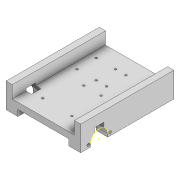
# Autodesk Inventor part: 본체판(구)
Saved by Autodesk Inventor 2020 (Build 240168000, 168)
## iProperties
Created: 2022-08-24
Part Number: 본체판(구)
Material: 일반
Document SubType Name: Modeling
Designer: 박연호
Density: 1 g/cm^3
Appearance: 기본값
Author: 박연호
Autodesk Inventor part; units mm, degrees
ref_plane "YZ Plane" through (0, 0, 0) normal (1, 0, 0) x (0, 1, 0)
ref_plane "XZ Plane" through (0, 0, 0) normal (0, 1, 0) x (-1, 0, 0)
ref_plane "XY Plane" through (0, 0, 0) normal (0, 0, 1) x (1, 0, 0)
sketch "스케치1" plane through (0, 0, 0) normal (0, 1, 0) x (-1, 0, 0)
  line L0 (60, 75) -> (-60, 75)
  line L1 (-60, 75) -> (-60, -75)
  line L2 (-60, -75) -> (60, -75)
  line L3 (60, -75) -> (60, 75)
  line L4 (60, 75) -> (-60, -75) construction
  line L5 (-60, 75) -> (60, -75) construction
  point P0 (0, 0)
  dimension "d0" = 120
  dimension "d1" = 150
  constraints: 12 end point, 2 midpoint, 2 parallel, 1 horizontal, 1 perpendicular
  measures "d0" distance of L0.start L0.end
  measures "d1" distance of L0.end L1.end
extrude "돌출1" add sketch "스케치1" along normal blind 40
sketch "스케치2" plane through (0, 40, 0) normal (0, 1, 0) x (1, 0, 0)
  line L0 (60, -75) -> (60, 75) projected
  line L1 (60, 75) -> (-60, 75) projected
  line L2 (50, 102.1646) -> (-50, 102.1646)
  line L3 (-50, 102.1646) -> (-50, -103.0725)
  line L4 (-50, -103.0725) -> (50, -103.0725)
  line L5 (50, -103.0725) -> (50, 102.1646)
  line L6 (-60, 75) -> (-60, -75) projected
  point P0 (0, 0)
  point P1 (50, 75)
  point P2 (-50, 75)
  dimension "d6" = 10
  dimension "d7" = 10
  constraints: 8 end point, 2 parallel, 1 horizontal, 1 perpendicular
  measures "d6" distance between parallel lines of L5 L0
  measures "d7" distance between parallel lines of L6 L3
extrude "돌출2" cut sketch "스케치2" against normal blind 20 contours L5 L4 L3 L1
sketch "스케치3" plane through (60, 0, 75) normal (1, 0, 0) x (0, 0, -1)
  circle A0 centre (29.6769, 5) radius 14
  circle A1 centre (120, 5) radius 14
  line L0 (150, 0) -> (150, 40) projected
  line L1 (0, 0) -> (150, 0) projected
  point P0 (75, 0)
  dimension "d10" = 28
  dimension "d12" = 28
  dimension "d13" = 30
  dimension "d16" = 5
  dimension "d30" = 5
  constraints: 2 centre point
  measures "d10" diameter of A0
  measures "d12" diameter of A1
  measures "d13" distance from line of L0 A1.centre
  measures "d16" distance from line of L1 A0.centre
  measures "d30" distance from line of L1 A1.centre
extrude "돌출3" cut sketch "스케치3" against normal blind 19 contours A0 L1 | L1 A0
sketch "스케치4" plane through (60, 0, -75) normal (1, 0, 0) x (0, 0, -1)
  arc A0 (-107.2464, 0) -> (-133.3998, 0) centre (-120.3231, 5) ccw projected
  line L0 (-134.3231, 36.9687) -> (-106.3231, 36.9687)
  line L1 (-106.3231, 36.9687) -> (-106.3231, -26.9687)
  line L2 (-106.3231, -26.9687) -> (-134.3231, -26.9687)
  line L3 (-134.3231, -26.9687) -> (-134.3231, 36.9687)
  line L4 (-134.3231, 36.9687) -> (-106.3231, -26.9687) construction
  line L5 (-106.3231, 36.9687) -> (-134.3231, -26.9687) construction
  line L6 (-150, 0) -> (-133.3998, 0) projected
  line L7 (-107.2464, 0) -> (0, 0) projected
  point P0 (-75, 0)
  point P1 (-134.3231, 0)
  point P2 (-134.3231, 5)
  point P3 (-106.3231, 0)
  point P4 (-106.3231, 5)
  dimension "d17" = 28
  constraints: 12 end point, 2 midpoint, 2 parallel, 1 horizontal, 1 perpendicular
  measures "d17" distance of L1.end L2.end
extrude "돌출4" cut sketch "스케치4" against normal blind 19 contours A0 L1 L7 | A0 L6 L3
sketch "스케치5" plane through (60, 0, -75) normal (1, 0, 0) x (0, 0, -1)
  line L0 (-127.8231, 12) -> (-112.8231, 12)
  line L1 (-112.8231, 12) -> (-112.8231, 24)
  line L2 (-112.8231, 24) -> (-127.8231, 24)
  line L3 (-127.8231, 24) -> (-127.8231, 12)
  line L4 (-127.8231, 12) -> (-112.8231, 24) construction
  line L5 (-112.8231, 12) -> (-127.8231, 24) construction
  arc A0 (-106.3231, 5) -> (-134.3231, 5) centre (-120.3231, 5) ccw projected
  point P0 (-75, 0)
  point P1 (-120.3231, 18)
  point P2 (-120.3231, 10)
  dimension "d20" = 15
  dimension "d32" = 19
  dimension "d33" = 0
  constraints: 12 end point, 2 midpoint, 2 parallel, 1 horizontal, 1 perpendicular
  measures "d20" distance of L1.end L2.end
  measures "d32" distance from line of L2 A0.centre
  measures "d33" horizontal distance of point (-120.323, 10) point (-120.323, 18)
extrude "돌출5" cut sketch "스케치5" against normal blind 19
sketch "스케치6" plane through (60, 0, -75) normal (1, 0, 0) x (0, 0, -1)
  arc A0 (-106.3231, 5) -> (-134.3231, 5) centre (-120.3231, 5) ccw projected
  point P0 (-75, 0)
  point P1 (-127.8231, 16.8216)
sketch "스케치7" plane through (60, 0, -75) normal (1, 0, 0) x (0, 0, -1)
  circle A0 centre (-120.3231, 5) radius 17.5 construction
  circle A1 centre (-102.8231, 5) radius 2.1
  circle A2 centre (-137.8231, 5) radius 2.1
  point P0 (-75, 0)
  dimension "d34" = 35
  dimension "d35" = 4.2
  dimension "d36" = 4.2
  constraints: 3 centre point, 2 point on circle, 1 coincident
  measures "d34" diameter of A0
  measures "d35" diameter of A1
  measures "d36" diameter of A2
extrude "돌출6" cut sketch "스케치7" against normal blind 19
mirror "미러1" about plane through (0, 0, 0) normal (1, 0, 0) of "돌출6", "돌출5", "돌출4", "돌출3"
sketch "스케치8" plane through (0, 0, 0) normal (0, -1, 0) x (1, 0, 0)
  line L0 (-41, -88.7468) -> (41, -88.7468)
  line L1 (41, -88.7468) -> (41, 88.7468)
  line L2 (41, 88.7468) -> (-41, 88.7468)
  line L3 (-41, 88.7468) -> (-41, -88.7468)
  line L4 (-41, -88.7468) -> (41, 88.7468) construction
  line L5 (41, -88.7468) -> (-41, 88.7468) construction
  line L6 (41, 31.3231) -> (41, 59.3231) projected
  point P0 (0, 0)
  dimension "d39" = 0
  constraints: 12 end point, 2 midpoint, 2 parallel, 1 horizontal, 1 perpendicular
  measures "d39" distance between parallel lines of L6 L1
extrude "돌출7" cut sketch "스케치8" against normal blind 10
sketch "스케치9" plane through (0, 20, 0) normal (0, 1, 0) x (1, 0, 0)
  line L0 (-28.9457, -65) -> (24.4543, -65)
  line L1 (24.4543, -65) -> (24.4543, 3.6)
  line L2 (24.4543, 3.6) -> (-28.9457, 3.6)
  line L3 (-28.9457, 3.6) -> (-28.9457, -65)
  line L4 (50, -75) -> (-50, -75) projected
  circle A0 centre (-26.3957, -49.7) radius 1.6
  circle A1 centre (21.9043, -51.03) radius 1.6
  circle A2 centre (16.8243, 1.05) radius 1.6
  circle A3 centre (-11.1057, 1.05) radius 1.6
  point P0 (0, 0)
  dimension "d42" = 53.4
  dimension "d43" = 68.6
  dimension "d44" = 10
  dimension "d45" = 3.2
  dimension "d46" = 15.3
  dimension "d47" = 2.55
  dimension "d51" = 3.2
  dimension "d52" = 2.55
  dimension "d56" = 13.97
  dimension "d57" = 3.2
  dimension "d58" = 7.63
  dimension "d59" = 2.55
  dimension "d60" = 3.2
  dimension "d61" = 2.55
  dimension "d62" = 35.56
  constraints: 8 end point, 4 centre point, 2 parallel, 1 horizontal, 1 perpendicular
  measures "d42" distance between parallel lines of L1 L3
  measures "d43" distance of L2.end L0.start
  measures "d44" distance between parallel lines of L0 L4
  measures "d45" diameter of A0
  measures "d46" distance from line of A0.centre L0
  measures "d47" distance from line of A0.centre L3
  measures "d51" diameter of A1
  measures "d52" distance from line of L1 A1.centre
  measures "d56" vertical distance of A1.centre L0.end
  measures "d57" diameter of A2
  measures "d58" distance from line of L1 A2.centre
  measures "d59" distance from line of L2 A2.centre
  measures "d60" diameter of A3
  measures "d61" distance from line of L2 A3.centre
  measures "d62" distance from line of A3.centre L1
extrude "돌출8" cut sketch "스케치9" against normal through all contours A0 | A1 | A2 | A3
sketch "스케치10" plane through (0, 20, 0) normal (0, 1, 0) x (1, 0, 0)
  line L0 (50, -75) -> (-50, -75) projected
  line L1 (2.7, 12.7) -> (45, 12.7)
  line L2 (45, 12.7) -> (45, 55)
  line L3 (45, 55) -> (2.7, 55)
  line L4 (2.7, 55) -> (2.7, 12.7)
  line L5 (-50, -75) -> (-50, 75) projected
  line L6 (50, 75) -> (50, -75) projected
  line L7 (39.35, 18.35) -> (8.35, 18.35)
  line L8 (8.35, 18.35) -> (8.35, 49.35)
  line L9 (8.35, 49.35) -> (39.35, 49.35)
  line L10 (39.35, 49.35) -> (39.35, 18.35)
  line L11 (39.35, 18.35) -> (8.35, 49.35) construction
  line L12 (8.35, 18.35) -> (39.35, 49.35) construction
  line L13 (-50, 75) -> (50, 75) projected
  circle A0 centre (8.35, 49.35) radius 1.6
  circle A1 centre (8.35, 18.35) radius 1.6
  circle A2 centre (39.35, 18.35) radius 1.6
  circle A3 centre (39.35, 49.35) radius 1.6
  point P0 (0, 0)
  point P1 (23.85, 33.85)
  dimension "d68" = 42.3
  dimension "d69" = 42.3
  dimension "d71" = 5
  dimension "d72" = 31
  dimension "d73" = 31
  dimension "d75" = 21.15
  dimension "d76" = 21.15
  dimension "d77" = 20
  dimension "d79" = 3.2
  dimension "d80" = 3.2
  dimension "d81" = 3.2
  dimension "d82" = 3.2
  constraints: 20 end point, 4 centre point, 4 coincident, 4 parallel, 2 horizontal, 2 midpoint, 2 perpendicular
  measures "d68" distance of L2.end L3.end
  measures "d69" distance of L3.end L1.start
  measures "d71" distance between parallel lines of L6 L2
  measures "d72" distance of L7.end L8.end
  measures "d73" distance of L8.end L9.end
  measures "d75" distance from line of L1 point (23.85, 33.85)
  measures "d76" distance from line of L4 point (23.85, 33.85)
  measures "d77" distance between parallel lines of L13 L3
  measures "d79" diameter of A0
  measures "d80" diameter of A1
  measures "d81" diameter of A2
  measures "d82" diameter of A3
extrude "돌출9" cut sketch "스케치10" against normal through all contours A1 L8 L7 | L7 L8 A1 | A2 L10 L7 | L7 L10 A2 | A0 L9 L8 | L8 L9 A0 | A3 L9 L10 | L10 L9 A3
mirror "미러2" about plane through (0, 0, 0) normal (1, 0, 0) of "돌출9"
